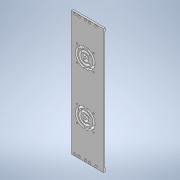
# Autodesk Inventor part: rIGHTbOXcOVER
Saved by Autodesk Inventor 2020 (Build 240168000, 168)
## iProperties
Created: 2019-06-04
Part Number: rIGHTbOXcOVER
Material: Generic
Document SubType Name: Modeling
Designer: LillaHunden
Density: 1 g/cm^3
Appearance: Default
Author: LillaHunden
Autodesk Inventor part; units mm, degrees
ref_plane "YZ Plane" through (0, 0, 0) normal (1, 0, 0) x (0, 1, 0)
ref_plane "XZ Plane" through (0, 0, 0) normal (0, 1, 0) x (-1, 0, 0)
ref_plane "XY Plane" through (0, 0, 0) normal (0, 0, 1) x (1, 0, 0)
sketch "Sketch1" plane through (0, 0, 0) normal (0, 0, 1) x (1, 0, 0)
  line L0 (19.3148, -120.8816) -> (20.6898, -123.2631) construction
  line L1 (20.6898, -123.2631) -> (23.4398, -123.2631) construction
  line L2 (23.4398, -123.2631) -> (24.8148, -120.8816) construction
  line L3 (24.8148, -120.8816) -> (23.4398, -118.5) construction
  line L4 (23.4398, -118.5) -> (20.6898, -118.5) construction
  line L5 (20.6898, -118.5) -> (19.3148, -120.8816) construction
  line L6 (13.4398, -123.2631) -> (14.8148, -120.8816) construction
  line L7 (14.8148, -120.8816) -> (13.4398, -118.5) construction
  line L8 (13.4398, -118.5) -> (10.6898, -118.5) construction
  line L9 (10.6898, -118.5) -> (9.3148, -120.8816) construction
  line L10 (9.3148, -120.8816) -> (10.6898, -123.2631) construction
  line L11 (10.6898, -123.2631) -> (13.4398, -123.2631) construction
  line L12 (15.6073, -115.6184) -> (14.2323, -118) construction
  line L13 (14.2323, -118) -> (15.6073, -120.3816) construction
  line L14 (15.6073, -120.3816) -> (18.3573, -120.3816) construction
  line L15 (18.3573, -120.3816) -> (19.7323, -118) construction
  line L16 (19.7323, -118) -> (18.3573, -115.6184) construction
  line L17 (18.3573, -115.6184) -> (15.6073, -115.6184) construction
  line L18 (24.2323, -112.2369) -> (25.6073, -114.6184) construction
  line L19 (25.6073, -114.6184) -> (28.3573, -114.6184) construction
  line L20 (28.3573, -114.6184) -> (29.7323, -112.2369) construction
  line L21 (29.7323, -112.2369) -> (28.3573, -109.8553) construction
  line L22 (28.3573, -109.8553) -> (25.6073, -109.8553) construction
  line L23 (25.6073, -109.8553) -> (24.2323, -112.2369) construction
  line L24 (13.4398, -124.2631) -> (10.6898, -124.2631) construction
  line L25 (10.6898, -124.2631) -> (9.3148, -126.6447) construction
  line L26 (9.3148, -126.6447) -> (10.6898, -129.0263) construction
  line L27 (10.6898, -129.0263) -> (13.4398, -129.0263) construction
  line L28 (13.4398, -129.0263) -> (14.8148, -126.6447) construction
  line L29 (14.8148, -126.6447) -> (13.4398, -124.2631) construction
  line L30 (25.6073, -126.1447) -> (28.3573, -126.1447) construction
  line L31 (28.3573, -126.1447) -> (29.7323, -123.7631) construction
  line L32 (29.7323, -123.7631) -> (28.3573, -121.3816) construction
  line L33 (28.3573, -121.3816) -> (25.6073, -121.3816) construction
  line L34 (25.6073, -121.3816) -> (24.2323, -123.7631) construction
  line L35 (24.2323, -123.7631) -> (25.6073, -126.1447) construction
  line L36 (19.3148, -115.1184) -> (20.6898, -117.5) construction
  line L37 (20.6898, -117.5) -> (23.4398, -117.5) construction
  line L38 (23.4398, -117.5) -> (24.8148, -115.1184) construction
  line L39 (24.8148, -115.1184) -> (23.4398, -112.7369) construction
  line L40 (23.4398, -112.7369) -> (20.6898, -112.7369) construction
  line L41 (20.6898, -112.7369) -> (19.3148, -115.1184) construction
  line L42 (10.6898, -117.5) -> (13.4398, -117.5) construction
  line L43 (13.4398, -117.5) -> (14.8148, -115.1184) construction
  line L44 (14.8148, -115.1184) -> (13.4398, -112.7369) construction
  line L45 (13.4398, -112.7369) -> (10.6898, -112.7369) construction
  line L46 (10.6898, -112.7369) -> (9.3148, -115.1184) construction
  line L47 (9.3148, -115.1184) -> (10.6898, -117.5) construction
  line L48 (24.2323, -118) -> (25.6073, -120.3816) construction
  line L49 (25.6073, -120.3816) -> (28.3573, -120.3816) construction
  line L50 (28.3573, -120.3816) -> (29.7323, -118) construction
  line L51 (29.7323, -118) -> (28.3573, -115.6184) construction
  line L52 (28.3573, -115.6184) -> (25.6073, -115.6184) construction
  line L53 (25.6073, -115.6184) -> (24.2323, -118) construction
  line L54 (14.2323, -123.7631) -> (15.6073, -126.1447) construction
  line L55 (15.6073, -126.1447) -> (18.3573, -126.1447) construction
  line L56 (18.3573, -126.1447) -> (19.7323, -123.7631) construction
  line L57 (19.7323, -123.7631) -> (18.3573, -121.3816) construction
  line L58 (18.3573, -121.3816) -> (15.6073, -121.3816) construction
  line L59 (15.6073, -121.3816) -> (14.2323, -123.7631) construction
  line L60 (19.7323, -112.2369) -> (18.3573, -109.8553) construction
  line L61 (18.3573, -109.8553) -> (15.6073, -109.8553) construction
  line L62 (15.6073, -109.8553) -> (14.2323, -112.2369) construction
  line L63 (14.2323, -112.2369) -> (15.6073, -114.6184) construction
  line L64 (15.6073, -114.6184) -> (18.3573, -114.6184) construction
  line L65 (18.3573, -114.6184) -> (19.7323, -112.2369) construction
  line L66 (20.6898, -124.2631) -> (19.3148, -126.6447) construction
  line L67 (19.3148, -126.6447) -> (20.6898, -129.0263) construction
  line L68 (20.6898, -129.0263) -> (23.4398, -129.0263) construction
  line L69 (23.4398, -129.0263) -> (24.8148, -126.6447) construction
  line L70 (24.8148, -126.6447) -> (23.4398, -124.2631) construction
  line L71 (23.4398, -124.2631) -> (20.6898, -124.2631) construction
  line L72 (0, -288) -> (0, 12) projected
  line L73 (0, 12) -> (76.9823, 12) projected
  line L74 (76.9823, 12) -> (76.9823, -288) projected
  line L75 (76.9823, -288) -> (0, -288) projected
  line L76 (44.8148, -137.8816) -> (43.4398, -135.5) projected
  line L77 (43.4398, -135.5) -> (40.6898, -135.5) projected
  line L78 (40.6898, -135.5) -> (39.3148, -137.8816) projected
  line L79 (39.3148, -137.8816) -> (40.6898, -140.2631) projected
  line L80 (40.6898, -140.2631) -> (43.4398, -140.2631) projected
  line L81 (43.4398, -140.2631) -> (44.8148, -137.8816) projected
  line L82 (44.8148, -143.6447) -> (43.4398, -141.2631) projected
  line L83 (43.4398, -141.2631) -> (40.6898, -141.2631) projected
  line L84 (40.6898, -141.2631) -> (39.3148, -143.6447) projected
  line L85 (39.3148, -143.6447) -> (40.6898, -146.0263) projected
  line L86 (40.6898, -146.0263) -> (43.4398, -146.0263) projected
  line L87 (43.4398, -146.0263) -> (44.8148, -143.6447) projected
  line L88 (34.2323, -129.2369) -> (35.6073, -131.6184) projected
  line L89 (35.6073, -131.6184) -> (38.3573, -131.6184) projected
  line L90 (38.3573, -131.6184) -> (39.7323, -129.2369) projected
  line L91 (39.7323, -129.2369) -> (38.3573, -126.8553) projected
  line L92 (38.3573, -126.8553) -> (35.6073, -126.8553) projected
  line L93 (35.6073, -126.8553) -> (34.2323, -129.2369) projected
  line L94 (38.3573, -138.3816) -> (35.6073, -138.3816) projected
  line L95 (35.6073, -138.3816) -> (34.2323, -140.7631) projected
  line L96 (34.2323, -140.7631) -> (35.6073, -143.1447) projected
  line L97 (35.6073, -143.1447) -> (38.3573, -143.1447) projected
  line L98 (38.3573, -143.1447) -> (39.7323, -140.7631) projected
  line L99 (39.7323, -140.7631) -> (38.3573, -138.3816) projected
  line L100 (49.7323, -135) -> (48.3573, -132.6184) projected
  line L101 (48.3573, -132.6184) -> (45.6073, -132.6184) projected
  line L102 (45.6073, -132.6184) -> (44.2323, -135) projected
  line L103 (44.2323, -135) -> (45.6073, -137.3816) projected
  line L104 (45.6073, -137.3816) -> (48.3573, -137.3816) projected
  line L105 (48.3573, -137.3816) -> (49.7323, -135) projected
  line L106 (30.6898, -129.7369) -> (29.3148, -132.1184) projected
  line L107 (29.3148, -132.1184) -> (30.6898, -134.5) projected
  line L108 (30.6898, -134.5) -> (33.4398, -134.5) projected
  line L109 (33.4398, -134.5) -> (34.8148, -132.1184) projected
  line L110 (34.8148, -132.1184) -> (33.4398, -129.7369) projected
  line L111 (33.4398, -129.7369) -> (30.6898, -129.7369) projected
  line L112 (44.8148, -132.1184) -> (43.4398, -129.7369) projected
  line L113 (43.4398, -129.7369) -> (40.6898, -129.7369) projected
  line L114 (40.6898, -129.7369) -> (39.3148, -132.1184) projected
  line L115 (39.3148, -132.1184) -> (40.6898, -134.5) projected
  line L116 (40.6898, -134.5) -> (43.4398, -134.5) projected
  line L117 (43.4398, -134.5) -> (44.8148, -132.1184) projected
  line L118 (45.6073, -138.3816) -> (44.2323, -140.7631) projected
  line L119 (44.2323, -140.7631) -> (45.6073, -143.1447) projected
  line L120 (45.6073, -143.1447) -> (48.3573, -143.1447) projected
  line L121 (48.3573, -143.1447) -> (49.7323, -140.7631) projected
  line L122 (49.7323, -140.7631) -> (48.3573, -138.3816) projected
  line L123 (48.3573, -138.3816) -> (45.6073, -138.3816) projected
  line L124 (30.6898, -146.0263) -> (33.4398, -146.0263) projected
  line L125 (33.4398, -146.0263) -> (34.8148, -143.6447) projected
  line L126 (34.8148, -143.6447) -> (33.4398, -141.2631) projected
  line L127 (33.4398, -141.2631) -> (30.6898, -141.2631) projected
  line L128 (30.6898, -141.2631) -> (29.3148, -143.6447) projected
  line L129 (29.3148, -143.6447) -> (30.6898, -146.0263) projected
  line L130 (48.3573, -126.8553) -> (45.6073, -126.8553) projected
  line L131 (45.6073, -126.8553) -> (44.2323, -129.2369) projected
  line L132 (44.2323, -129.2369) -> (45.6073, -131.6184) projected
  line L133 (45.6073, -131.6184) -> (48.3573, -131.6184) projected
  line L134 (48.3573, -131.6184) -> (49.7323, -129.2369) projected
  line L135 (49.7323, -129.2369) -> (48.3573, -126.8553) projected
  line L136 (38.3573, -137.3816) -> (39.7323, -135) projected
  line L137 (39.7323, -135) -> (38.3573, -132.6184) projected
  line L138 (38.3573, -132.6184) -> (35.6073, -132.6184) projected
  line L139 (35.6073, -132.6184) -> (34.2323, -135) projected
  line L140 (34.2323, -135) -> (35.6073, -137.3816) projected
  line L141 (35.6073, -137.3816) -> (38.3573, -137.3816) projected
  line L142 (29.3148, -137.8816) -> (30.6898, -140.2631) projected
  line L143 (30.6898, -140.2631) -> (33.4398, -140.2631) projected
  line L144 (33.4398, -140.2631) -> (34.8148, -137.8816) projected
  line L145 (34.8148, -137.8816) -> (33.4398, -135.5) projected
  line L146 (33.4398, -135.5) -> (30.6898, -135.5) projected
  line L147 (30.6898, -135.5) -> (29.3148, -137.8816) projected
  line L148 (24.8148, -137.8816) -> (23.4398, -135.5) projected
  line L149 (23.4398, -135.5) -> (20.6898, -135.5) projected
  line L150 (20.6898, -135.5) -> (19.3148, -137.8816) projected
  line L151 (19.3148, -137.8816) -> (20.6898, -140.2631) projected
  line L152 (20.6898, -140.2631) -> (23.4398, -140.2631) projected
  line L153 (23.4398, -140.2631) -> (24.8148, -137.8816) projected
  line L154 (24.8148, -143.6447) -> (23.4398, -141.2631) projected
  line L155 (23.4398, -141.2631) -> (20.6898, -141.2631) projected
  line L156 (20.6898, -141.2631) -> (19.3148, -143.6447) projected
  line L157 (19.3148, -143.6447) -> (20.6898, -146.0263) projected
  line L158 (20.6898, -146.0263) -> (23.4398, -146.0263) projected
  line L159 (23.4398, -146.0263) -> (24.8148, -143.6447) projected
  line L160 (14.2323, -129.2369) -> (15.6073, -131.6184) projected
  line L161 (15.6073, -131.6184) -> (18.3573, -131.6184) projected
  line L162 (18.3573, -131.6184) -> (19.7323, -129.2369) projected
  line L163 (19.7323, -129.2369) -> (18.3573, -126.8553) projected
  line L164 (18.3573, -126.8553) -> (15.6073, -126.8553) projected
  line L165 (15.6073, -126.8553) -> (14.2323, -129.2369) projected
  line L166 (18.3573, -138.3816) -> (15.6073, -138.3816) projected
  line L167 (15.6073, -138.3816) -> (14.2323, -140.7631) projected
  line L168 (14.2323, -140.7631) -> (15.6073, -143.1447) projected
  line L169 (15.6073, -143.1447) -> (18.3573, -143.1447) projected
  line L170 (18.3573, -143.1447) -> (19.7323, -140.7631) projected
  line L171 (19.7323, -140.7631) -> (18.3573, -138.3816) projected
  line L172 (29.7323, -135) -> (28.3573, -132.6184) projected
  line L173 (28.3573, -132.6184) -> (25.6073, -132.6184) projected
  line L174 (25.6073, -132.6184) -> (24.2323, -135) projected
  line L175 (24.2323, -135) -> (25.6073, -137.3816) projected
  line L176 (25.6073, -137.3816) -> (28.3573, -137.3816) projected
  line L177 (28.3573, -137.3816) -> (29.7323, -135) projected
  line L178 (10.6898, -129.7369) -> (9.3148, -132.1184) projected
  line L179 (9.3148, -132.1184) -> (10.6898, -134.5) projected
  line L180 (10.6898, -134.5) -> (13.4398, -134.5) projected
  line L181 (13.4398, -134.5) -> (14.8148, -132.1184) projected
  line L182 (14.8148, -132.1184) -> (13.4398, -129.7369) projected
  line L183 (13.4398, -129.7369) -> (10.6898, -129.7369) projected
  line L184 (24.8148, -132.1184) -> (23.4398, -129.7369) projected
  line L185 (23.4398, -129.7369) -> (20.6898, -129.7369) projected
  line L186 (20.6898, -129.7369) -> (19.3148, -132.1184) projected
  line L187 (19.3148, -132.1184) -> (20.6898, -134.5) projected
  line L188 (20.6898, -134.5) -> (23.4398, -134.5) projected
  line L189 (23.4398, -134.5) -> (24.8148, -132.1184) projected
  line L190 (25.6073, -138.3816) -> (24.2323, -140.7631) projected
  line L191 (24.2323, -140.7631) -> (25.6073, -143.1447) projected
  line L192 (25.6073, -143.1447) -> (28.3573, -143.1447) projected
  line L193 (28.3573, -143.1447) -> (29.7323, -140.7631) projected
  line L194 (29.7323, -140.7631) -> (28.3573, -138.3816) projected
  line L195 (28.3573, -138.3816) -> (25.6073, -138.3816) projected
  line L196 (10.6898, -146.0263) -> (13.4398, -146.0263) projected
  line L197 (13.4398, -146.0263) -> (14.8148, -143.6447) projected
  line L198 (14.8148, -143.6447) -> (13.4398, -141.2631) projected
  line L199 (13.4398, -141.2631) -> (10.6898, -141.2631) projected
  line L200 (10.6898, -141.2631) -> (9.3148, -143.6447) projected
  line L201 (9.3148, -143.6447) -> (10.6898, -146.0263) projected
  line L202 (28.3573, -126.8553) -> (25.6073, -126.8553) projected
  line L203 (25.6073, -126.8553) -> (24.2323, -129.2369) projected
  line L204 (24.2323, -129.2369) -> (25.6073, -131.6184) projected
  line L205 (25.6073, -131.6184) -> (28.3573, -131.6184) projected
  line L206 (28.3573, -131.6184) -> (29.7323, -129.2369) projected
  line L207 (29.7323, -129.2369) -> (28.3573, -126.8553) projected
  line L208 (18.3573, -137.3816) -> (19.7323, -135) projected
  line L209 (19.7323, -135) -> (18.3573, -132.6184) projected
  line L210 (18.3573, -132.6184) -> (15.6073, -132.6184) projected
  line L211 (15.6073, -132.6184) -> (14.2323, -135) projected
  line L212 (14.2323, -135) -> (15.6073, -137.3816) projected
  line L213 (15.6073, -137.3816) -> (18.3573, -137.3816) projected
  line L214 (9.3148, -137.8816) -> (10.6898, -140.2631) projected
  line L215 (10.6898, -140.2631) -> (13.4398, -140.2631) projected
  line L216 (13.4398, -140.2631) -> (14.8148, -137.8816) projected
  line L217 (14.8148, -137.8816) -> (13.4398, -135.5) projected
  line L218 (13.4398, -135.5) -> (10.6898, -135.5) projected
  line L219 (10.6898, -135.5) -> (9.3148, -137.8816) projected
  line L220 (44.8148, -120.8816) -> (43.4398, -118.5) projected
  line L221 (43.4398, -118.5) -> (40.6898, -118.5) projected
  line L222 (40.6898, -118.5) -> (39.3148, -120.8816) projected
  line L223 (39.3148, -120.8816) -> (40.6898, -123.2631) projected
  line L224 (40.6898, -123.2631) -> (43.4398, -123.2631) projected
  line L225 (43.4398, -123.2631) -> (44.8148, -120.8816) projected
  line L226 (44.8148, -126.6447) -> (43.4398, -124.2631) projected
  line L227 (43.4398, -124.2631) -> (40.6898, -124.2631) projected
  line L228 (40.6898, -124.2631) -> (39.3148, -126.6447) projected
  line L229 (39.3148, -126.6447) -> (40.6898, -129.0263) projected
  line L230 (40.6898, -129.0263) -> (43.4398, -129.0263) projected
  line L231 (43.4398, -129.0263) -> (44.8148, -126.6447) projected
  line L232 (34.2323, -112.2369) -> (35.6073, -114.6184) projected
  line L233 (35.6073, -114.6184) -> (38.3573, -114.6184) projected
  line L234 (38.3573, -114.6184) -> (39.7323, -112.2369) projected
  line L235 (39.7323, -112.2369) -> (38.3573, -109.8553) projected
  line L236 (38.3573, -109.8553) -> (35.6073, -109.8553) projected
  line L237 (35.6073, -109.8553) -> (34.2323, -112.2369) projected
  line L238 (38.3573, -121.3816) -> (35.6073, -121.3816) projected
  line L239 (35.6073, -121.3816) -> (34.2323, -123.7631) projected
  line L240 (34.2323, -123.7631) -> (35.6073, -126.1447) projected
  line L241 (35.6073, -126.1447) -> (38.3573, -126.1447) projected
  line L242 (38.3573, -126.1447) -> (39.7323, -123.7631) projected
  line L243 (39.7323, -123.7631) -> (38.3573, -121.3816) projected
  line L244 (49.7323, -118) -> (48.3573, -115.6184) projected
  line L245 (48.3573, -115.6184) -> (45.6073, -115.6184) projected
  line L246 (45.6073, -115.6184) -> (44.2323, -118) projected
  line L247 (44.2323, -118) -> (45.6073, -120.3816) projected
  line L248 (45.6073, -120.3816) -> (48.3573, -120.3816) projected
  line L249 (48.3573, -120.3816) -> (49.7323, -118) projected
  line L250 (30.6898, -112.7369) -> (29.3148, -115.1184) projected
  line L251 (29.3148, -115.1184) -> (30.6898, -117.5) projected
  line L252 (30.6898, -117.5) -> (33.4398, -117.5) projected
  line L253 (33.4398, -117.5) -> (34.8148, -115.1184) projected
  line L254 (34.8148, -115.1184) -> (33.4398, -112.7369) projected
  line L255 (33.4398, -112.7369) -> (30.6898, -112.7369) projected
  line L256 (44.8148, -115.1184) -> (43.4398, -112.7369) projected
  line L257 (43.4398, -112.7369) -> (40.6898, -112.7369) projected
  line L258 (40.6898, -112.7369) -> (39.3148, -115.1184) projected
  line L259 (39.3148, -115.1184) -> (40.6898, -117.5) projected
  line L260 (40.6898, -117.5) -> (43.4398, -117.5) projected
  line L261 (43.4398, -117.5) -> (44.8148, -115.1184) projected
  line L262 (45.6073, -121.3816) -> (44.2323, -123.7631) projected
  line L263 (44.2323, -123.7631) -> (45.6073, -126.1447) projected
  line L264 (45.6073, -126.1447) -> (48.3573, -126.1447) projected
  line L265 (48.3573, -126.1447) -> (49.7323, -123.7631) projected
  line L266 (49.7323, -123.7631) -> (48.3573, -121.3816) projected
  line L267 (48.3573, -121.3816) -> (45.6073, -121.3816) projected
  line L268 (30.6898, -129.0263) -> (33.4398, -129.0263) projected
  line L269 (33.4398, -129.0263) -> (34.8148, -126.6447) projected
  line L270 (34.8148, -126.6447) -> (33.4398, -124.2631) projected
  line L271 (33.4398, -124.2631) -> (30.6898, -124.2631) projected
  line L272 (30.6898, -124.2631) -> (29.3148, -126.6447) projected
  line L273 (29.3148, -126.6447) -> (30.6898, -129.0263) projected
  line L274 (48.3573, -109.8553) -> (45.6073, -109.8553) projected
  line L275 (45.6073, -109.8553) -> (44.2323, -112.2369) projected
  line L276 (44.2323, -112.2369) -> (45.6073, -114.6184) projected
  line L277 (45.6073, -114.6184) -> (48.3573, -114.6184) projected
  line L278 (48.3573, -114.6184) -> (49.7323, -112.2369) projected
  line L279 (49.7323, -112.2369) -> (48.3573, -109.8553) projected
  line L280 (38.3573, -120.3816) -> (39.7323, -118) projected
  line L281 (39.7323, -118) -> (38.3573, -115.6184) projected
  line L282 (38.3573, -115.6184) -> (35.6073, -115.6184) projected
  line L283 (35.6073, -115.6184) -> (34.2323, -118) projected
  line L284 (34.2323, -118) -> (35.6073, -120.3816) projected
  line L285 (35.6073, -120.3816) -> (38.3573, -120.3816) projected
  line L286 (29.3148, -120.8816) -> (30.6898, -123.2631) projected
  line L287 (30.6898, -123.2631) -> (33.4398, -123.2631) projected
  line L288 (33.4398, -123.2631) -> (34.8148, -120.8816) projected
  line L289 (34.8148, -120.8816) -> (33.4398, -118.5) projected
  line L290 (33.4398, -118.5) -> (30.6898, -118.5) projected
  line L291 (30.6898, -118.5) -> (29.3148, -120.8816) projected
  circle A0 centre (18, -283.95) radius 3.15 projected
  circle A1 centre (43.4912, -283.95) radius 3.15 projected
  circle A2 centre (68.9823, -283.95) radius 3.15 projected
  circle A3 centre (58.9823, -283.95) radius 3.15 projected
  circle A4 centre (33.4912, -283.95) radius 3.15 projected
  circle A5 centre (8, -283.95) radius 3.15 projected
  circle A6 centre (18, 7.95) radius 3.15 projected
  circle A7 centre (43.4912, 7.95) radius 3.15 projected
  circle A8 centre (68.9823, 7.95) radius 3.15 projected
  circle A9 centre (33.4912, 7.95) radius 3.15 projected
  circle A10 centre (8, 7.95) radius 3.15 projected
  circle A11 centre (58.9823, 7.95) radius 3.15 projected
  circle A12 centre (51.5, -236.7541) radius 3.15 projected
  circle A13 centre (51.5, -186.7541) radius 3.15 projected
  circle A14 centre (61.5, -161.7541) radius 3.15 projected
  circle A15 centre (61.5, -186.7541) radius 3.15 projected
  circle A16 centre (61.5, -211.7541) radius 3.15 projected
  circle A17 centre (51.5, -161.7541) radius 3.15 projected
  circle A18 centre (51.5, -211.7541) radius 3.15 projected
  circle A19 centre (51.5, -261.7541) radius 3.15 projected
  point P0 (0, 0)
extrude "Extrusion1" add sketch "Sketch1" along normal blind 12 contours L72 L73 L74 L75 | L81 L80 L79 L78 L77 L76 | L87 L86 L85 L84 L83 L82 | L93 L92 L91 L90 L89 L88 | L99 L98 L97 L96 L95 L94 | L105 L104 L103 L102 L101 L100 | L111 L110 L109 L108 L107 L106 | L117 L116 L115 L114 L113 L112 | L123 L122 L121 L120 L119 L118 | L129 L128 L127 L126 L125 L124 | L135 L134 L133 L132 L131 L130 | L141 L140 L139 L138 L137 L136 | L147 L146 L145 L144 L143 L142 | L153 L152 L151 L150 L149 L148 | L159 L158 L157 L156 L155 L154 | L165 L164 L163 L162 L161 L160 | L171 L170 L169 L168 L167 L166 | L177 L176 L175 L174 L173 L172 | L183 L182 L181 L180 L179 L178 | L189 L188 L187 L186 L185 L184 | L195 L194 L193 L192 L191 L190 | L201 L200 L199 L198 L197 L196 | L207 L206 L205 L204 L203 L202 | L213 L212 L211 L210 L209 L208 | L219 L218 L217 L216 L215 L214 | L225 L224 L223 L222 L221 L220 | L231 L230 L229 L228 L227 L226 | L237 L236 L235 L234 L233 L232 | L243 L242 L241 L240 L239 L238 | L249 L248 L247 L246 L245 L244 | L255 L254 L253 L252 L251 L250 | L261 L260 L259 L258 L257 L256 | L267 L266 L265 L264 L263 L262 | L273 L272 L271 L270 L269 L268 | L279 L278 L277 L276 L275 L274 | L285 L284 L283 L282 L281 L280 | L291 L290 L289 L288 L287 L286 | A0 | A1 | A2 | A3 | A4 | A5 | A6 | A7 | A8 | A9 | A10 | A11 | A12 | A13 | A14 | A15 | A16 | A17 | A18 | A19
sketch "Sketch2" plane through (0, 0, 0) normal (0, 0, -1) x (-1, 0, 0)
  line L0 (-67, 4) -> (-76.9823, 4) construction
  line L1 (-76.9823, -280) -> (-76.9823, 4) construction
  line L2 (-67, -280) -> (-76.9823, -280) construction
  line L3 (-67, 4) -> (-67, -280) construction
  line L4 (-66.8, -280.2) -> (-77.1823, -280.2)
  line L5 (-77.1823, -280.2) -> (-77.1823, 4.2)
  line L6 (-77.1823, 4.2) -> (-66.8, 4.2)
  line L7 (-66.8, 4.2) -> (-66.8, -280.2)
  point P0 (0, 0)
  dimension "d2" = 0.2
  constraints: 8 end point, 3 other
  measures "d2" distance between parallel lines of L3 L7
extrude "Extrusion2" cut sketch "Sketch2" against normal blind 9.25
sketch "Sketch3" plane through (0, 0, 0) normal (0, 0, -1) x (-1, 0, 0)
  line L0 (0, -276) -> (-67, -276) construction
  line L1 (-76.9823, -288) -> (0, -288) construction
  line L2 (-76.9823, -280) -> (-76.9823, -288) construction
  line L3 (-67, -280) -> (-67, 4) construction
  line L4 (-76.9823, -288) -> (0, -288)
  line L5 (0, -288) -> (0, -275.8)
  line L6 (0, -275.8) -> (-76.9823, -275.8)
  line L7 (-76.9823, -275.8) -> (-76.9823, -288)
  line L8 (0, 12) -> (0, -288) projected
  point P0 (0, 0)
  point P1 (0, -281.9)
  dimension "d5" = 0.2
  constraints: 8 end point, 2 parallel, 1 horizontal, 1 midpoint, 1 perpendicular, 1 point on line
  measures "d5" distance between parallel lines of L0 L6
extrude "Extrusion3" cut sketch "Sketch3" against normal blind 8.05
sketch "Sketch4" plane through (66.8, -280.2, 9.25) normal (1, 0, 0) x (0, 0, -1)
  line L0 (1.2, 4.4) -> (9.25, 4.4) construction
  line L1 (9.25, 284.4) -> (9.25, 4.4) construction
  line L2 (9.25, 284.4) -> (0, 284.4) projected
  line L3 (0, 284.4) -> (0, 0) projected
  line L4 (1.2, 0) -> (0, 0) projected
  line L5 (1.2, 0) -> (1.2, 4.4) projected
  line L6 (1.25, 284.2) -> (1.25, 0.2) projected
  line L7 (1.25, 284.2) -> (1.25, 284.4)
  line L8 (0, 284.4) -> (1.2, 284.4)
  line L9 (1.2, 284.4) -> (1.2, 0)
  line L10 (1.2, 0) -> (0, 0)
  line L11 (0, 0) -> (0, 284.4)
  point P0 (9.25, 280.2)
  constraints: 10 end point, 2 parallel, 2 perpendicular, 1 horizontal, 1 point on line
extrude "Extrusion4" add sketch "Sketch4" along normal blind 9
sketch "Sketch5" plane through (0, 0, 0) normal (0, 0, -1) x (-1, 0, 0)
  line L0 (0, 0) -> (-67, 0) construction
  line L1 (-75.8, 4.2) -> (-66.8, 4.2) construction
  line L2 (-66.8, 4.2) -> (-66.8, -275.8) construction
  line L3 (-76.9823, 4.2) -> (-66.8, 4.2) construction
  line L4 (-76.9823, 4.2) -> (-76.9823, 12) construction
  line L5 (-76.9823, 12) -> (0, 12) construction
  line L6 (0, 12) -> (0, -275.8) construction
  line L7 (0, -0.2) -> (-67, -0.2)
  line L8 (-76.9823, 12) -> (0, 12)
  line L9 (0, 12) -> (0, -0.2)
  line L10 (0, -0.2) -> (-76.9823, -0.2)
  line L11 (-76.9823, -0.2) -> (-76.9823, 12)
  dimension "d10" = 0.2
  constraints: 10 end point, 3 parallel, 1 horizontal, 1 perpendicular
  measures "d10" distance between parallel lines of L0 L7
ref_plane "Work Plane1" through (0, 0, 8) normal (0, 0, 1) x (1, 0, 0)
extrude "Extrusion5" cut sketch "Sketch5" against normal up to surface (8 mm away)
sketch "Sketch6" plane through (0, -0.2, 0) normal (0, 1, 0) x (1, 0, 0)
  point P0 (56.9823, -3)
  point P1 (46.9823, -3)
  point P2 (30, -3)
  point P3 (20, -3)
hole "Hole1" at (56.9823, -0.2, 3) at (46.9823, -0.2, 3) at (30, -0.2, 3) at (20, -0.2, 3) direction (0, -1, 0) diameter 2.459 depth 8 tip angle 120 thread size "M3x0.5" class "6H" standard "ISO Metric profile"
sketch "Sketch7" plane through (0, 0, 12) normal (0, 0, 1) x (1, 0, 0)
  circle A0 centre (68.9823, 7.95) radius 3.15 construction
  circle A1 centre (58.9823, 7.95) radius 3.15 construction
  circle A2 centre (43.4912, 7.95) radius 3.15 construction
  circle A3 centre (33.4912, 7.95) radius 3.15 construction
  circle A4 centre (18, 7.95) radius 3.15 construction
  circle A5 centre (8, 7.95) radius 3.15 construction
  circle A6 centre (8, -283.95) radius 3.15 construction
  circle A7 centre (18, -283.95) radius 3.15 construction
  circle A8 centre (33.4912, -283.95) radius 3.15 construction
  circle A9 centre (43.4912, -283.95) radius 3.15 construction
  circle A10 centre (58.9823, -283.95) radius 3.15 construction
  circle A11 centre (68.9823, -283.95) radius 3.15 construction
  point P0 (0, 0)
sketch "Sketch9" plane through (0, 0, 12) normal (0, 0, 1) x (1, 0, 0)
  point P0 (8, 7.95)
  point P1 (18, 7.95)
  point P2 (33.4912, 7.95)
  point P3 (43.4912, 7.95)
  point P4 (58.9823, 7.95)
hole "Hole4" at (8, 7.95, 12) at (18, 7.95, 12) at (33.4912, 7.95, 12) at (43.4912, 7.95, 12) at (58.9823, 7.95, 12) direction (0, 0, -1) diameter 3.4 depth 4 countersink diameter 6.3 countersink angle 90
sketch "Sketch10" plane through (0, 0, 12) normal (0, 0, 1) x (1, 0, 0)
  point P0 (58.9823, -283.95)
  point P1 (43.4912, -283.95)
  point P2 (33.4912, -283.95)
  point P3 (18, -283.95)
  point P4 (8, -283.95)
hole "Hole6" at (58.9823, -283.95, 12) at (43.4912, -283.95, 12) at (33.4912, -283.95, 12) at (18, -283.95, 12) at (8, -283.95, 12) direction (0, 0, -1) diameter 3.4 depth 3.95 countersink diameter 6.3 countersink angle 90
sketch "Sketch11" plane through (0, 0, 12) normal (0, 0, 1) x (1, 0, 0)
  line L0 (53, -176.5677) -> (13, -176.5677) construction
  line L1 (13, -176.5677) -> (13, -216.5677) construction
  line L2 (13, -216.5677) -> (53, -216.5677) construction
  line L3 (53, -216.5677) -> (53, -176.5677) construction
  line L4 (53, -50.8348) -> (13, -50.8348) construction
  line L5 (13, -50.8348) -> (13, -90.8348) construction
  line L6 (13, -90.8348) -> (53, -90.8348) construction
  line L7 (53, -90.8348) -> (53, -50.8348) construction
  line L8 (0, 12) -> (0, -288) projected
  point P0 (0, 0)
  point P1 (53, -70.8348)
  point P2 (53, -196.5677)
  dimension "d41" = 40
  dimension "d42" = 40
  dimension "d43" = 40
  dimension "d44" = 40
  dimension "d45" = 13
  constraints: 16 end point, 8 coincident, 4 parallel, 2 horizontal, 2 midpoint, 2 perpendicular, 1 vertical alignment
  measures "d41" distance of L2.end L1.end
  measures "d42" distance of L1.end L0.end
  measures "d43" distance of L6.end L5.end
  measures "d44" distance of L5.end L4.end
  measures "d45" distance between parallel lines of L8 L5
hole "Hole8" at (13, -176.5677, 12) at (13, -216.5677, 12) at (53, -216.5677, 12) at (53, -176.5677, 12) at (13, -50.8348, 12) at (13, -90.8348, 12) at (53, -90.8348, 12) at (53, -50.8348, 12) direction (0, 0, -1) diameter 3.242 end through all thread size "M4x0.7" class "6H" standard "ISO Metric profile"
sketch "Sketch12" plane through (0, 0, 12) normal (0, 0, 1) x (1, 0, 0)
  circle A0 centre (53, -90.8348) radius 1.621 construction
  circle A1 centre (13, -50.8348) radius 1.621 construction
  circle A2 centre (53, -216.5677) radius 1.621 construction
  circle A3 centre (13, -176.5677) radius 1.621 construction
  circle A4 centre (13, -216.5677) radius 1.621 construction
  circle A5 centre (53, -176.5677) radius 1.621 construction
  circle A6 centre (13, -90.8348) radius 1.621 construction
  circle A7 centre (53, -50.8348) radius 1.621 construction
  circle A8 centre (18, -283.95) radius 3.15 construction
  circle A9 centre (43.4912, -283.95) radius 3.15 construction
  circle A10 centre (58.9823, -283.95) radius 3.15 construction
  circle A11 centre (33.4912, -283.95) radius 3.15 construction
  circle A12 centre (8, -283.95) radius 3.15 construction
  circle A13 centre (43.4912, 7.95) radius 3.15 construction
  circle A14 centre (18, 7.95) radius 3.15 construction
  circle A15 centre (8, 7.95) radius 3.15 construction
  circle A16 centre (33.4912, 7.95) radius 3.15 construction
  circle A17 centre (58.9823, 7.95) radius 3.15 construction
  line L0 (76.9823, 12) -> (0, 12) construction
  line L1 (0, 12) -> (0, -288) construction
  line L2 (0, -288) -> (76.9823, -288) construction
  line L3 (76.9823, -288) -> (76.9823, 12) construction
  line L4 (53, -90.8348) -> (13, -50.8348) construction
  line L5 (13, -50.8348) -> (53, -50.8348) construction
  line L6 (53, -50.8348) -> (13, -90.8348) construction
  line L7 (13, -176.5677) -> (13, -216.5677) construction
  line L8 (13, -216.5677) -> (53, -216.5677) construction
  line L9 (53, -216.5677) -> (13, -176.5677) construction
  line L10 (53, -176.5677) -> (13, -216.5677) construction
  circle A18 centre (33, -70.8348) radius 24 construction
  circle A19 centre (33, -196.5677) radius 24 construction
  arc A20 (37.3584, -91.5413) -> (37.3584, -50.1283) centre (33, -70.8348) ccw construction
  arc A21 (37.8806, -94.0225) -> (37.8806, -47.647) centre (33, -70.8348) ccw
  arc A22 (36.8361, -89.06) -> (36.8361, -52.6095) centre (33, -70.8348) ccw
  arc A23 (36.8361, -89.06) -> (37.8806, -94.0225) centre (37.3584, -91.5413) ccw
  arc A24 (37.8806, -47.647) -> (36.8361, -52.6095) centre (37.3584, -50.1283) ccw
  arc A25 (42.3123, -61.5224) -> (42.3123, -80.1471) centre (33, -70.8348) ccw construction
  arc A26 (44.1052, -59.7295) -> (44.1052, -81.94) centre (33, -70.8348) ccw
  arc A27 (40.5194, -63.3154) -> (40.5194, -78.3541) centre (33, -70.8348) ccw
  arc A28 (40.5194, -63.3154) -> (44.1052, -59.7295) centre (42.3123, -61.5224) ccw
  arc A29 (44.1052, -81.94) -> (40.5194, -78.3541) centre (42.3123, -80.1471) ccw
  line L11 (33, -43.5046) -> (33, -109.6187) construction
  line L12 (53, -50.8348) -> (13, -50.8348) construction
  circle A30 centre (33, -70.8348) radius 24 construction
  arc A31 (28.6416, -50.1283) -> (28.6416, -91.5413) centre (33, -70.8348) ccw construction
  arc A32 (28.1194, -47.647) -> (28.1194, -94.0225) centre (33, -70.8348) ccw
  arc A33 (29.1639, -52.6095) -> (29.1639, -89.06) centre (33, -70.8348) ccw
  arc A34 (28.1194, -94.0225) -> (29.1639, -89.06) centre (28.6416, -91.5413) ccw
  arc A35 (29.1639, -52.6095) -> (28.1194, -47.647) centre (28.6416, -50.1283) ccw
  arc A36 (30.3412, -75.5506) -> (30.3412, -66.1189) centre (33, -70.8348) ccw construction
  arc A37 (29.0751, -77.7962) -> (29.0751, -63.8734) centre (33, -70.8348) ccw
  arc A38 (31.6072, -73.3051) -> (31.6072, -68.3644) centre (33, -70.8348) ccw
  arc A39 (31.6072, -73.3051) -> (29.0751, -77.7962) centre (30.3412, -75.5506) ccw
  arc A40 (29.0751, -63.8734) -> (31.6072, -68.3644) centre (30.3412, -66.1189) ccw
  arc A41 (28.1194, -219.7555) -> (29.1639, -214.793) centre (28.6416, -217.2743) ccw
  arc A42 (44.1052, -207.673) -> (40.5194, -204.0871) centre (42.3123, -205.8801) ccw
  arc A43 (29.0751, -203.5292) -> (29.0751, -189.6064) centre (33, -196.5678) ccw
  arc A44 (29.0751, -189.6064) -> (31.6072, -194.0974) centre (30.3412, -191.8519) ccw
  arc A45 (40.5194, -189.0484) -> (40.5194, -204.0871) centre (33, -196.5678) ccw
  arc A46 (37.8806, -173.38) -> (36.8361, -178.3425) centre (37.3584, -175.8613) ccw
  arc A47 (42.3123, -187.2554) -> (42.3123, -205.8801) centre (33, -196.5678) ccw construction
  arc A48 (29.1639, -178.3425) -> (28.1194, -173.38) centre (28.6416, -175.8613) ccw
  arc A49 (36.8361, -214.793) -> (36.8361, -178.3425) centre (33, -196.5678) ccw
  arc A50 (44.1052, -185.4625) -> (44.1052, -207.673) centre (33, -196.5678) ccw
  arc A51 (37.3584, -217.2743) -> (37.3584, -175.8613) centre (33, -196.5678) ccw construction
  arc A52 (29.1639, -178.3425) -> (29.1639, -214.793) centre (33, -196.5678) ccw
  arc A53 (37.8806, -219.7555) -> (37.8806, -173.38) centre (33, -196.5678) ccw
  line L13 (13, -176.5678) -> (53, -176.5678) construction
  line L14 (53, -176.5678) -> (13, -176.5678) construction
  line L15 (53, -216.5678) -> (13, -176.5678) construction
  line L16 (53, -176.5678) -> (13, -216.5678) construction
  circle A54 centre (33, -196.5678) radius 24 construction
  circle A55 centre (33, -196.5678) radius 24 construction
  arc A56 (28.6416, -175.8613) -> (28.6416, -217.2743) centre (33, -196.5678) ccw construction
  arc A57 (28.1194, -173.38) -> (28.1194, -219.7555) centre (33, -196.5678) ccw
  arc A58 (40.5194, -189.0484) -> (44.1052, -185.4625) centre (42.3123, -187.2554) ccw
  arc A59 (31.6072, -199.0381) -> (31.6072, -194.0974) centre (33, -196.5678) ccw
  arc A60 (30.3412, -201.2836) -> (30.3412, -191.8519) centre (33, -196.5678) ccw construction
  arc A61 (31.6072, -199.0381) -> (29.0751, -203.5292) centre (30.3412, -201.2836) ccw
  arc A62 (36.8361, -214.793) -> (37.8806, -219.7555) centre (37.3584, -217.2743) ccw
  point P0 (0, 0)
  point P1 (33, -169.2376)
  dimension "d53" = 48
  dimension "d54" = 48
  dimension "d55" = 2.5356
  dimension "d56" = 2.5356
  dimension "d59" = 125.733
  dimension "d62" = 125.733
  constraints: 80 point on circle, 45 centre point, 26 end point, 12 tangent, 8 coincident, 8 symmetric about line, 4 vertical alignment, 3 perpendicular, 3 vertical, 2 midpoint, 2 point on line, 1 horizontal, 67 other
  measures "d53" diameter of A18
  measures "d54" diameter of A19
  measures "d55" radius of A29
  measures "d56" radius of A23
  measures "d59" distance of A18.centre A19.centre
  measures "d62" distance of A34.centre A41.centre
extrude "Extrusion6" cut sketch "Sketch12" against normal through all
sketch "Sketch13" plane through (0, 0, 0) normal (0, 0, -1) x (-1, 0, 0)
  line L0 (-58, -98.3348) -> (-8, -98.3348)
  line L1 (-5.5, -95.8348) -> (-5.5, -45.8348)
  line L2 (-8, -43.3348) -> (-58, -43.3348)
  line L3 (-60.5, -45.8348) -> (-60.5, -95.8348)
  arc A0 (-31.6072, -68.3644) -> (-31.6072, -73.3051) centre (-33, -70.8348) ccw construction
  arc A1 (-60.5, -95.8348) -> (-58, -98.3348) centre (-58, -95.8348) ccw
  arc A2 (-58, -43.3348) -> (-60.5, -45.8348) centre (-58, -45.8348) ccw
  arc A3 (-5.5, -45.8348) -> (-8, -43.3348) centre (-8, -45.8348) ccw
  arc A4 (-8, -98.3348) -> (-5.5, -95.8348) centre (-8, -95.8348) ccw
  line L4 (-33, -70.8348) -> (-50.7028, -70.8348) construction
  arc A5 (-8, -224.0678) -> (-5.5, -221.5678) centre (-8, -221.5678) ccw
  line L5 (-58, -224.0678) -> (-8, -224.0678)
  arc A6 (-60.5, -221.5678) -> (-58, -224.0678) centre (-58, -221.5678) ccw
  line L6 (-5.5, -221.5678) -> (-5.5, -171.5678)
  line L7 (-33, -196.5678) -> (-50.7028, -196.5678) construction
  arc A7 (-5.5, -171.5678) -> (-8, -169.0678) centre (-8, -171.5678) ccw
  line L8 (-8, -169.0678) -> (-58, -169.0678)
  line L9 (-60.5, -171.5678) -> (-60.5, -221.5678)
  arc A8 (-58, -169.0678) -> (-60.5, -171.5678) centre (-58, -171.5678) ccw
  point P0 (0, 0)
  point P1 (-5.5, -43.3348)
  point P2 (-5.5, -98.3348)
  point P3 (-60.5, -43.3348)
  point P4 (-60.5, -70.8348)
  point P5 (-33, -43.3348)
  point P6 (-5.5, -224.0678)
  point P7 (-31.6072, -199.0381)
  point P8 (-31.6072, -194.0974)
  point P9 (-5.5, -169.0678)
  point P10 (-33, -169.0678)
  point P11 (-60.5, -169.0678)
  point P12 (-60.5, -196.5678)
  dimension "d67" = 55
  dimension "d68" = 55
  dimension "d69" = 2.5
  dimension "d72" = 125.733
  constraints: 20 end point, 16 point on circle, 12 point on line, 8 centre point, 8 tangent, 3 equal radius, 2 horizontal, 2 midpoint, 2 parallel, 1 collinear, 1 horizontal alignment, 1 perpendicular, 1 vertical, 1 vertical alignment, 29 other
  measures "d67" distance of point (-5.5, -43.335) point (-60.5, -43.335)
  measures "d68" distance of point (-5.5, -98.335) point (-5.5, -43.335)
  measures "d69" radius of A1
  measures "d72" distance of L1.start L6.start
extrude "Extrusion7" cut sketch "Sketch13" against normal blind 4.75
move faces "Move1" translate (0, 0, -0.05) faces at (72.8, -183.9333, 8.05)
equation "\"d56\" = d55"
equation "\"d68\" = d67"
body "Solid1"
